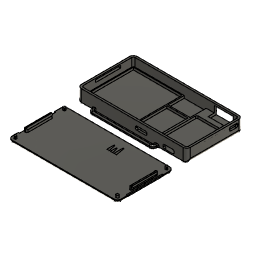
ArcturusV3 v8 (Autodesk Fusion 360 design; units mm, degrees)
Autodesk Fusion 360 part; units mm, degrees
(part 1 of 2)
sketch "Sketch8" plane through (0, 0, 0) normal (0, 0, 1) x (1, 0, 0)
  line L0 (45.1, 23.3) -> (-45.1, 23.3)
  line L1 (-45.1, -23.3) -> (45.1, -23.3)
  line L2 (45.1, -23.3) -> (45.1, 23.3)
  line L3 (45.1, 23.3) -> (-45.1, -23.3) construction
  line L4 (-45.1, 23.3) -> (45.1, -23.3) construction
  line L5 (-45.1, 23.3) -> (-46.1, 23.3)
  line L6 (-46.1, 23.3) -> (-46.1, -23.3)
  line L7 (-46.1, -23.3) -> (-45.1, -23.3)
  dimension "d32" = 90.2
  dimension "d33" = 46.6
  dimension "d223" = 1
  constraint horizontal L0
  constraint parallel L0 L1
  constraint coincident L3 origin
  constraint coincident L4 origin
  constraint horizontal L5
  constraint vertical L6
  constraint horizontal L7
  measures "d32" distance of L1.start L1.end
  measures "d33" distance of L0.end L1.start
  measures "d223" distance of L0.end L5.end
extrude "Extrude7" add sketch "Sketch8" along normal blind 10 makes body 1
fillet "Fillet4" radius 3 6 edges at (45.1, -23.3, 5) (45.1, 0, 0) (45.1, 23.3, 5) (-46.1, 23.3, 5) (-46.1, 0, 0) (-46.1, -23.3, 5) on bodies 1
sketch "Sketch13" plane through (0, 0, 10) normal (0, 0, 1) x (-1, 0, 0)
  line L0 (43.1, 23.3) -> (-42.1, 23.3)
  arc A0 (-42.1, 23.3) -> (-45.1, 20.3) centre (-42.1, 20.3) ccw
  line L1 (-45.1, 20.3) -> (-45.1, -20.3)
  arc A1 (-45.1, -20.3) -> (-42.1, -23.3) centre (-42.1, -20.3) ccw
  line L2 (-42.1, -23.3) -> (43.1, -23.3)
  line L3 (46.1, -20.3) -> (46.1, 20.3)
  arc A2 (46.1, 20.3) -> (43.1, 23.3) centre (43.1, 20.3) ccw
  arc A3 (43.1, -23.3) -> (46.1, -20.3) centre (43.1, -20.3) ccw
  line L4 (-43.5, 20.3) -> (-43.5, -20.3)
  arc A4 (-43.5, -20.3) -> (-42.1, -21.7) centre (-42.1, -20.3) ccw
  line L5 (-42.1, -21.7) -> (43.1, -21.7)
  arc A5 (43.1, -21.7) -> (44.5, -20.3) centre (43.1, -20.3) ccw
  line L6 (44.5, -20.3) -> (44.5, 20.3)
  arc A6 (44.5, 20.3) -> (43.1, 21.7) centre (43.1, 20.3) ccw
  line L7 (43.1, 21.7) -> (-42.1, 21.7)
  arc A7 (-42.1, 21.7) -> (-43.5, 20.3) centre (-42.1, 20.3) ccw
  dimension "d276" = -1.6
extrude "Extrude8" cut sketch "Sketch13" against normal blind 6 contours L4 A4 L5 A5 L6 A6 L7 A7 bodies 1
sketch "Sketch17" plane through (0, 0, 4) normal (0, 0, 1) x (-1, 0, 0)
  line L0 (1.989, 21.7) -> (-15.811, 21.7)
  line L1 (-15.811, 21.7) -> (-15.811, -6.1)
  line L2 (-14.811, -7.1) -> (0.989, -7.1)
  line L3 (1.989, -6.1) -> (1.989, 21.7)
  line L4 (1.989, -6.1) -> (1.989, -7.1)
  line L5 (1.989, -7.1) -> (0.989, -7.1)
  line L6 (-14.811, -7.1) -> (-15.811, -7.1)
  line L7 (-15.811, -6.1) -> (-15.811, -7.1)
  arc A0 (-42.1, 21.7) -> (-43.5, 20.3) centre (-42.1, 20.3) ccw
  line L8 (-43.5, 20.3) -> (-43.5, -20.3)
  arc A1 (-43.5, -20.3) -> (-42.1, -21.7) centre (-42.1, -20.3) ccw
  line L9 (-42.1, -21.7) -> (43.1, -21.7)
  arc A2 (43.1, -21.7) -> (44.5, -20.3) centre (43.1, -20.3) ccw
  line L10 (44.5, -20.3) -> (44.5, 20.3)
  arc A3 (44.5, 20.3) -> (43.1, 21.7) centre (43.1, 20.3) ccw
  line L11 (43.1, 21.7) -> (-42.1, 21.7)
  point P0 (1.989, -7.1)
  point P1 (43.1, -21.1)
  point P2 (43.1, -21.3)
  point P3 (43.1, -21.3)
  dimension "d53" = 17.8
  dimension "d54" = 28.8
  constraint horizontal L0
  constraint vertical L1
  constraint horizontal L2
  constraint vertical L3
  constraint coincident P0 L2
  constraint coincident P0 L3
  constraint coincident P0 L4.end
  constraint perpendicular L1 L6
  constraint perpendicular L6 L7
  measures "d53" distance of L0.start L0.end
  measures "d54" distance of L0.start P0
extrude "Extrude10" cut sketch "Sketch17" against normal blind 2 contours L0 L1 L2 L3 L4 L5 L6 L7 L11 bodies 1
sketch "Sketch20" plane through (0, 0, 4) normal (0, 0, 1) x (-1, 0, 0)
  line L0 (1.989, 21.7) -> (1.989, -7.1)
  line L1 (1.989, -7.1) -> (-15.811, -7.1)
  line L2 (-15.811, -7.1) -> (-15.811, 21.7)
  line L3 (-15.811, 21.7) -> (-42.1, 21.7)
  line L4 (43.1, 21.7) -> (1.989, 21.7)
  line L5 (1, -8) -> (-15.4, -8)
  line L6 (-16.4, -9) -> (-16.4, -21.4)
  line L7 (-16.4, -21.4) -> (2, -21.4)
  line L8 (2, -21.4) -> (2, -9)
  line L9 (-16.4, -9) -> (-16.4, -8)
  line L10 (-15.4, -8) -> (-16.4, -8)
  line L11 (1, -8) -> (2, -8)
  line L12 (2, -9) -> (2, -8)
  arc A0 (-42.1, 21.7) -> (-43.5, 20.3) centre (-42.1, 20.3) ccw
  line L13 (-43.5, 20.3) -> (-43.5, -20.3)
  arc A1 (-43.5, -20.3) -> (-42.1, -21.7) centre (-42.1, -20.3) ccw
  line L14 (-42.1, -21.7) -> (43.1, -21.7)
  arc A2 (43.1, -21.7) -> (44.5, -20.3) centre (43.1, -20.3) ccw
  line L15 (44.5, -20.3) -> (44.5, 20.3)
  arc A3 (44.5, 20.3) -> (43.1, 21.7) centre (43.1, 20.3) ccw
  point P0 (2, -8)
  point P1 (-16.4, -8)
  dimension "d61" = 18.4
  dimension "d62" = 13.4
  constraint horizontal L5
  constraint vertical L6
  constraint horizontal L7
  constraint vertical L8
  constraint coincident P1 L5
  constraint coincident P1 L6
  constraint coincident P0 L5
  constraint coincident P0 L8
  constraint coincident P1 L9.end
  constraint coincident P0 L11.end
  measures "d61" distance of P0 P1
  measures "d62" distance of P0 L7.end
extrude "Extrude11" cut sketch "Sketch20" against normal blind 2 contours L5 L6 L7 L8 L9 L10 L11 L12 bodies 1
sketch "Sketch24" plane through (0, 0, 4) normal (0, 0, 1) x (-1, 0, 0)
  line L0 (-16.4, -8) -> (2, -8)
  line L1 (2, -8) -> (2, -21.4)
  line L2 (2, -21.4) -> (-16.4, -21.4)
  line L3 (-16.4, -21.4) -> (-16.4, -8)
  line L4 (1.989, 21.7) -> (1.989, -7.1)
  line L5 (1.989, -7.1) -> (-15.811, -7.1)
  line L6 (-15.811, -7.1) -> (-15.811, 21.7)
  line L7 (-15.811, 21.7) -> (-42.1, 21.7)
  line L8 (43.1, 21.7) -> (1.989, 21.7)
  line L9 (4, 21) -> (43.5, 21)
  line L10 (43.5, 21) -> (43.5, -21)
  line L11 (43.5, -21) -> (4, -21)
  line L12 (3, -20) -> (3, 20)
  arc A0 (4, 21) -> (3, 20) centre (4, 20) ccw
  arc A1 (3, -20) -> (4, -21) centre (4, -20) ccw
  arc A2 (-42.1, 21.7) -> (-43.5, 20.3) centre (-42.1, 20.3) ccw
  line L13 (-43.5, 20.3) -> (-43.5, -20.3)
  arc A3 (-43.5, -20.3) -> (-42.1, -21.7) centre (-42.1, -20.3) ccw
  line L14 (-42.1, -21.7) -> (43.1, -21.7)
  arc A4 (43.1, -21.7) -> (44.5, -20.3) centre (43.1, -20.3) ccw
  line L15 (44.5, -20.3) -> (44.5, 20.3)
  arc A5 (44.5, 20.3) -> (43.1, 21.7) centre (43.1, 20.3) ccw
  point P0 (3, 21)
  point P1 (3, -21)
  dimension "d67" = 40.5
  dimension "d68" = 42
  dimension "d97" = 1
  constraint horizontal L9
  constraint vertical L10
  constraint horizontal L11
  constraint vertical L12
  constraint coincident P0 L9
  constraint coincident P0 L12
  constraint tangent L9 A0
  constraint tangent L12 A0
  constraint coincident P1 L11
  constraint coincident P1 L12
  constraint tangent L11 A1
  constraint tangent L12 A1
  constraint equal A0 A1
  measures "d67" distance of P0 L9.end
  measures "d68" distance of P0 P1
  measures "d97" radius of A0
extrude "Extrude12" cut sketch "Sketch24" against normal blind 2 contours L9 L10 L11 L12 A0 A1 bodies 1
sketch "Sketch26" plane through (0, 0, 4) normal (0, 0, 1) x (-1, 0, 0)
  line L0 (43.5, -21) -> (4, -21)
  line L1 (3, -20) -> (3, 20)
  line L2 (4, 21) -> (43.5, 21)
  line L3 (43.5, 21) -> (43.5, -21)
  line L4 (-15.811, 21.7) -> (-42.1, 21.7)
  line L5 (1.989, 21.7) -> (1.989, -7.1)
  line L6 (1.989, -7.1) -> (-15.811, -7.1)
  line L7 (-15.811, -7.1) -> (-15.811, 21.7)
  line L8 (-16.4, -8) -> (2, -8)
  line L9 (2, -8) -> (2, -21.4)
  line L10 (2, -21.4) -> (-16.4, -21.4)
  line L11 (-16.4, -21.4) -> (-16.4, -8)
  line L12 (-17.533, 21.7) -> (-42.933, 21.7)
  line L13 (-42.933, 21.7) -> (-42.933, -12.7)
  line L14 (-41.933, -13.7) -> (-18.533, -13.7)
  line L15 (-17.533, -12.7) -> (-17.533, 21.7)
  arc A0 (-18.533, -13.7) -> (-17.533, -12.7) centre (-18.533, -12.7) ccw
  arc A1 (-42.933, -12.7) -> (-41.933, -13.7) centre (-41.933, -12.7) ccw
  arc A2 (3, -20) -> (4, -21) centre (4, -20) ccw
  arc A3 (4, 21) -> (3, 20) centre (4, 20) ccw
  arc A4 (-42.1, 21.7) -> (-43.5, 20.3) centre (-42.1, 20.3) ccw
  line L16 (-43.5, 20.3) -> (-43.5, -20.3)
  arc A5 (-43.5, -20.3) -> (-42.1, -21.7) centre (-42.1, -20.3) ccw
  line L17 (-42.1, -21.7) -> (43.1, -21.7)
  arc A6 (43.1, -21.7) -> (44.5, -20.3) centre (43.1, -20.3) ccw
  line L18 (44.5, -20.3) -> (44.5, 20.3)
  arc A7 (44.5, 20.3) -> (43.1, 21.7) centre (43.1, 20.3) ccw
  line L19 (43.1, 21.7) -> (1.989, 21.7)
  point P0 (-17.533, -13.7)
  dimension "d73" = 25.4
  dimension "d74" = 35.4
  dimension "d94" = 1
  constraint horizontal L12
  constraint vertical L13
  constraint horizontal L14
  constraint vertical L15
  constraint coincident P0 L14
  constraint coincident P0 L15
  constraint tangent L14 A0
  constraint tangent L15 A0
  constraint tangent L13 A1
  constraint tangent L14 A1
  constraint equal A0 A1
  measures "d73" distance of L12.start L12.end
  measures "d74" distance of L12.start P0
  measures "d94" radius of A0
extrude "Extrude13" cut sketch "Sketch26" against normal blind 2 contours L4 L12 L13 L14 L15 A0 A1 A4 | L12 L13 A4 bodies 1
sketch "Sketch29" plane through (0, 0, 4) normal (0, 0, 1) x (-1, 0, 0)
  line L0 (-16.4, -8) -> (2, -8)
  line L1 (2, -8) -> (2, -21.4)
  line L2 (2, -21.4) -> (-16.4, -21.4)
  line L3 (-16.4, -21.4) -> (-16.4, -8)
  line L4 (-17.533, 21.7) -> (-17.533, -12.7)
  line L5 (-18.533, -13.7) -> (-41.933, -13.7)
  line L6 (-42.933, -12.7) -> (-42.933, 21.4252)
  line L7 (43.5, -21) -> (4, -21)
  line L8 (3, -20) -> (3, 20)
  line L9 (4, 21) -> (43.5, 21)
  line L10 (43.5, 21) -> (43.5, -21)
  line L11 (43.1, 21.7) -> (1.989, 21.7)
  line L12 (1.989, 21.7) -> (1.989, -7.1)
  line L13 (1.989, -7.1) -> (-15.811, -7.1)
  line L14 (-15.811, -7.1) -> (-15.811, 21.7)
  line L15 (-15.811, 21.7) -> (-17.533, 21.7)
  line L16 (-39.0432, -21.7) -> (-23.2432, -21.7)
  line L17 (-23.2432, -21.7) -> (-23.2432, -15.5)
  line L18 (-23.2432, -15.5) -> (-39.0432, -15.5)
  line L19 (-39.0432, -15.5) -> (-39.0432, -21.7)
  arc A0 (-18.533, -13.7) -> (-17.533, -12.7) centre (-18.533, -12.7) ccw
  arc A1 (-42.933, -12.7) -> (-41.933, -13.7) centre (-41.933, -12.7) ccw
  arc A2 (3, -20) -> (4, -21) centre (4, -20) ccw
  arc A3 (4, 21) -> (3, 20) centre (4, 20) ccw
  arc A4 (-42.933, 21.4252) -> (-43.5, 20.3) centre (-42.1, 20.3) ccw
  line L20 (-43.5, 20.3) -> (-43.5, -20.3)
  arc A5 (-43.5, -20.3) -> (-42.1, -21.7) centre (-42.1, -20.3) ccw
  line L21 (-42.1, -21.7) -> (43.1, -21.7)
  arc A6 (43.1, -21.7) -> (44.5, -20.3) centre (43.1, -20.3) ccw
  line L22 (44.5, -20.3) -> (44.5, 20.3)
  arc A7 (44.5, 20.3) -> (43.1, 21.7) centre (43.1, 20.3) ccw
  dimension "d81" = 15.8
  dimension "d82" = 6.2
  constraint horizontal L16
  constraint vertical L17
  constraint horizontal L18
  constraint vertical L19
  measures "d81" distance of L16.start L16.end
  measures "d82" distance of L16.start L18.end
extrude "Extrude14" cut sketch "Sketch29" against normal blind 2 contours L16 L17 L18 L19 L21 bodies 1
move_face "MoveFace1" by (0, -0.1, 0) 1 faces at (10.2667, 21.4, 3.3333) on bodies 1
move_face "MoveFace2" by (0, 0.3, 0) 1 faces at (10.2667, 21.3, 3.3333) on bodies 1
move_face "MoveFace3" by (0, 0.1, 0) 1 faces at (10.2667, 21.6, 3.3333) on bodies 1
sketch "Sketch31" plane through (0, 21.7, 0) normal (0, -1, 0) x (1, 0, 0)
  line L0 (-2, 4) -> (-2, 2)
  line L1 (-2, 2) -> (16.4, 2)
  line L2 (16.4, 2) -> (16.4, 4)
  line L3 (16.4, 4) -> (23.2432, 4)
  line L4 (23.2432, 4) -> (23.2432, 2)
  line L5 (23.2432, 2) -> (39.0432, 2)
  line L6 (39.0432, 2) -> (39.0432, 4)
  line L7 (39.0432, 4) -> (42.1, 4)
  line L8 (42.1, 10) -> (-43.1, 10)
  line L9 (23.2432, 2) -> (39.0432, 2)
  line L10 (39.0432, 2) -> (39.0432, 9.65)
  line L11 (39.0432, 9.65) -> (23.2432, 9.65)
  line L12 (23.2432, 9.65) -> (23.2432, 2)
  line L13 (42.1, 4) -> (42.1, 10)
  line L14 (-43.1, 10) -> (-43.1, 4)
  line L15 (-43.1, 4) -> (-2, 4)
  dimension "d85" = 15.8
  dimension "d86" = 7.65
  constraint horizontal L9
  constraint vertical L10
  constraint horizontal L11
  constraint vertical L12
  constraint coincident L4.end L5.start
  measures "d85" distance of L4.end L5.end
  measures "d86" distance of L4.end L11.end
extrude "Extrude15" cut sketch "Sketch31" against normal blind 2 contours L4 L5 L6 L9 L10 L11 L12 bodies 1
sketch "Sketch32" plane through (0, -21.7, 0) normal (0, 1, 0) x (-1, 0, 0)
  line L0 (43.1, 10) -> (-42.1, 10)
  line L1 (-42.933, 2) -> (-17.533, 2)
  line L2 (-17.533, 2) -> (-17.533, 4)
  line L3 (-17.533, 4) -> (-15.811, 4)
  line L4 (-15.811, 4) -> (-15.811, 2)
  line L5 (-15.811, 2) -> (1.989, 2)
  line L6 (1.989, 2) -> (1.989, 4)
  line L7 (1.989, 4) -> (43.1, 4)
  line L8 (-10.7121, 4.0287) -> (-3.2121, 4.0287)
  line L9 (-2.2121, 5.0287) -> (-2.2121, 6.0287)
  line L10 (-3.2121, 7.0287) -> (-10.7121, 7.0287)
  line L11 (-11.7121, 6.0287) -> (-11.7121, 5.0287)
  arc A0 (-10.7121, 7.0287) -> (-11.7121, 6.0287) centre (-10.7121, 6.0287) ccw
  arc A1 (-2.2121, 6.0287) -> (-3.2121, 7.0287) centre (-3.2121, 6.0287) ccw
  arc A2 (-3.2121, 4.0287) -> (-2.2121, 5.0287) centre (-3.2121, 5.0287) ccw
  arc A3 (-11.7121, 5.0287) -> (-10.7121, 4.0287) centre (-10.7121, 5.0287) ccw
  line L12 (-42.1, 10) -> (-42.1, 4)
  line L13 (-42.1, 4) -> (-42.933, 4)
  line L14 (-42.933, 4) -> (-42.933, 2)
  line L15 (43.1, 4) -> (43.1, 10)
  point P0 (-11.7121, 4.0287)
  point P1 (-2.2121, 4.0287)
  point P2 (-11.7121, 7.0287)
  dimension "d89" = 9.5
  dimension "d90" = 3
  dimension "d91" = 1
  constraint horizontal L8
  constraint vertical L9
  constraint horizontal L10
  constraint vertical L11
  constraint coincident P2 L10
  constraint coincident P2 L11
  constraint tangent L10 A0
  constraint tangent L11 A0
  constraint tangent L9 A1
  constraint tangent L10 A1
  constraint equal A0 A1
  constraint coincident P1 L8
  constraint coincident P1 L9
  constraint tangent L8 A2
  constraint tangent L9 A2
  constraint equal A0 A2
  constraint coincident P0 L8
  constraint coincident P0 L11
  constraint tangent L8 A3
  constraint tangent L11 A3
  constraint equal A0 A3
  measures "d89" distance of P0 P1
  measures "d90" distance of P0 P2
  measures "d91" radius of A0
extrude "Extrude16" cut sketch "Sketch32" against normal blind 2 contours L8 L9 L10 L11 A0 A1 A2 A3 bodies 1
sketch "Sketch33" plane through (0, -21.7, 0) normal (0, 1, 0) x (-1, 0, 0)
  line L0 (-3.2121, 4.0287) -> (-10.7121, 4.0287)
  arc A0 (-11.7121, 5.0287) -> (-10.7121, 4.0287) centre (-10.7121, 5.0287) ccw
  line L1 (-11.7121, 5.0287) -> (-11.7121, 6.0287)
  arc A1 (-10.7121, 7.0287) -> (-11.7121, 6.0287) centre (-10.7121, 6.0287) ccw
  line L2 (-10.7121, 7.0287) -> (-3.2121, 7.0287)
  arc A2 (-2.2121, 6.0287) -> (-3.2121, 7.0287) centre (-3.2121, 6.0287) ccw
  line L3 (-2.2121, 6.0287) -> (-2.2121, 5.0287)
  arc A3 (-3.2121, 4.0287) -> (-2.2121, 5.0287) centre (-3.2121, 5.0287) ccw
  line L4 (43.1, 10) -> (-42.1, 10)
  line L5 (-42.933, 2) -> (-17.533, 2)
  line L6 (-17.533, 2) -> (-17.533, 4)
  line L7 (-17.533, 4) -> (-15.811, 4)
  line L8 (-15.811, 4) -> (-15.811, 2)
  line L9 (-15.811, 2) -> (1.989, 2)
  line L10 (1.989, 2) -> (1.989, 4)
  line L11 (1.989, 4) -> (43.1, 4)
  line L12 (-33.5451, 2) -> (-26.3451, 2)
  line L13 (-25.3451, 3) -> (-25.3451, 4.2)
  line L14 (-26.3451, 5.2) -> (-33.5451, 5.2)
  line L15 (-34.5451, 4.2) -> (-34.5451, 3)
  arc A4 (-33.5451, 5.2) -> (-34.5451, 4.2) centre (-33.5451, 4.2) ccw
  arc A5 (-25.3451, 4.2) -> (-26.3451, 5.2) centre (-26.3451, 4.2) ccw
  arc A6 (-26.3451, 2) -> (-25.3451, 3) centre (-26.3451, 3) ccw
  arc A7 (-34.5451, 3) -> (-33.5451, 2) centre (-33.5451, 3) ccw
  line L16 (-42.1, 10) -> (-42.1, 4)
  line L17 (-42.1, 4) -> (-42.933, 4)
  line L18 (-42.933, 4) -> (-42.933, 2)
  line L19 (43.1, 4) -> (43.1, 10)
  point P0 (-34.5451, 2)
  point P1 (-25.3451, 2)
  point P2 (-34.5451, 5.2)
  dimension "d98" = 9.2
  dimension "d99" = 3.2
  dimension "d100" = 1
  dimension "d101" = 1
  constraint horizontal L12
  constraint vertical L13
  constraint horizontal L14
  constraint vertical L15
  constraint coincident L5 P0
  constraint coincident P2 L14
  constraint coincident P2 L15
  constraint tangent L14 A4
  constraint tangent L15 A4
  constraint tangent L13 A5
  constraint tangent L14 A5
  constraint coincident P1 L12
  constraint coincident P1 L13
  constraint tangent L12 A6
  constraint tangent L13 A6
  constraint equal A5 A6
  constraint coincident P0 L12
  constraint coincident P0 L15
  constraint tangent L12 A7
  constraint tangent L15 A7
  constraint equal A5 A7
  measures "d98" distance of P0 P1
  measures "d99" distance of P0 P2
  measures "d100" radius of A4
  measures "d101" radius of A5
extrude "Extrude17" cut sketch "Sketch33" against normal blind 2 contours L5 L12 L13 L14 L15 A4 A5 A6 A7 bodies 1
sketch "Sketch36" plane through (0, 0, 0) normal (0, 0, 1) x (1, 0, 0)
  line L0 (-33, -23) -> (-33, -24.5)
  line L1 (-30, -27.5) -> (18, -27.5)
  line L2 (21, -24.5) -> (21, -23)
  line L3 (-33, -23) -> (21, -23)
  arc A0 (18, -27.5) -> (21, -24.5) centre (18, -24.5) ccw
  arc A1 (-33, -24.5) -> (-30, -27.5) centre (-30, -24.5) ccw
  line L4 (21, -24.5) -> (21, -23)
  line L5 (21, -23) -> (18, -23)
  point P0 (21, -27.5)
  dimension "d111" = 3
  constraint vertical L0
  constraint horizontal L1
  constraint vertical L2
  constraint coincident P0 L1
  constraint coincident P0 L2
  constraint tangent L1 A0
  constraint tangent L2 A0
  constraint tangent L0 A1
  constraint tangent L1 A1
  constraint equal A0 A1
  constraint vertical L4
  constraint horizontal L5
  measures "d111" radius of A0
extrude "Extrude1" add sketch "Sketch36" along normal blind 3 separate body makes body 2 in component "Component"
sketch "Sketch38" plane through (0, 0, 3) normal (0, 0, 1) x (-1, 0, 0)
  line L0 (33, 23) -> (33, 24.5)
  arc A0 (33, 24.5) -> (30, 27.5) centre (30, 24.5) ccw
  line L1 (30, 27.5) -> (-18, 27.5)
  arc A1 (-18, 27.5) -> (-21, 24.5) centre (-18, 24.5) ccw
  line L2 (-21, 24.5) -> (-21, 23)
  line L3 (-21, 23) -> (33, 23)
  line L4 (30, 25.5) -> (-17.866, 25.5)
  line L5 (30.866, 24.5) -> (30.866, 23)
  line L6 (30.866, 23) -> (-18.866, 23)
  line L7 (-18.866, 23) -> (-18.866, 24.5)
  line L8 (-17.866, 25.5) -> (29.866, 25.5)
  line L9 (-18.866, 24.5) -> (-18.866, 23)
  arc A2 (-17.866, 25.5) -> (-18.866, 24.5) centre (-17.866, 24.5) ccw
  line L10 (30.866, 24.5) -> (30.866, 23)
  arc A3 (30.866, 24.5) -> (29.866, 25.5) centre (29.866, 24.5) ccw
  dimension "d273" = 1
  dimension "d274" = 1
  constraint vertical L5
  constraint horizontal L6
  constraint vertical L7
  constraint coincident L3 L5.end
  constraint tangent L9 A2
  constraint tangent L8 A2
  constraint perpendicular L6 L10
  constraint tangent L8 A3
  constraint tangent L5 A3
  measures "d273" radius of A2
  measures "d274" radius of A3
extrude "Extrude3" cut sketch "Sketch38" against normal blind 3 contours L3 L4 L5 L6 L7 L8 L9 A2 L10 A3 bodies 2 in component "Component"
combine "Combine2" operation add target body 1 tool bodies 2 2 body 2 seen with x (1, 0, 0) y (0, 1, 0) z (0, 0, 1) at (0, 0, 0) body 2 seen with x (-1, 0, 0) y (0, -1, 0) z (0, 0, 1) at (-12, 0, 0)
move_face "MoveFace4" by (0, 0, 1) 1 faces at (-14.7, 22.7667, 10) on bodies 1
sketch "Sketch40" plane through (43.5, 0, 0) normal (-1, 0, 0) x (0, -1, 0)
  line L0 (-18.5, 9) -> (-13.5, 9)
  line L1 (-12.5, 8) -> (-12.5, 7)
  line L2 (-13.5, 6) -> (-18.5, 6)
  line L3 (-19.5, 7) -> (-19.5, 8)
  arc A0 (-18.5, 9) -> (-19.5, 8) centre (-18.5, 8) ccw
  arc A1 (-13.5, 6) -> (-12.5, 7) centre (-13.5, 7) ccw
  arc A2 (-12.5, 8) -> (-13.5, 9) centre (-13.5, 8) ccw
  arc A3 (-19.5, 7) -> (-18.5, 6) centre (-18.5, 7) ccw
  line L4 (20.3, 11) -> (-20.3, 11)
  line L5 (-20.3, 11) -> (-20.3, 4)
  line L6 (-20.3, 4) -> (20.3, 4)
  line L7 (20.3, 4) -> (20.3, 11)
  dimension "d121" = 1
  constraint horizontal L0
  constraint vertical L1
  constraint horizontal L2
  constraint vertical L3
  constraint tangent L0 A0
  constraint tangent L3 A0
  constraint tangent L1 A1
  constraint tangent L2 A1
  constraint equal A0 A1
  constraint tangent L0 A2
  constraint tangent L1 A2
  constraint equal A0 A2
  constraint tangent L2 A3
  constraint tangent L3 A3
  constraint equal A0 A3
  measures "d121" radius of A0
extrude "Extrude18" cut sketch "Sketch40" against normal blind 2 contours L0 L1 L2 L3 A0 A1 A2 A3 bodies 1
fillet "Fillet6" radius 1 32 edges at (44.2213, 22.4213, 0.8787) (31.55, 23.3, 0) (21, 23.9, 0) (20.1213, 26.6213, 0) (-6, 27.5, 0) (-32.1213, 26.6213, 0) (-33, 23.9, 0) (21, 23.9, 3) (20.1213, 26.6213, 3) (-6, 27.5, 3) (-32.1213, 26.6213, 3) (-33, 23.9, 3) (-33, 23.3, 1.5) (21, 23.3, 1.5) (-38.05, 23.3, 0) (-45.2213, 22.4213, 0.8787) (-45.2213, -22.4213, 0.8787) (-38.05, -23.3, 0) (-33, -23.3, 1.5) (-33, -23.9, 0) (-32.1213, -26.6213, 0) (-6, -27.5, 0) (20.1213, -26.6213, 0) (21, -23.9, 0) (-33, -23.9, 3) (-32.1213, -26.6213, 3) (-6, -27.5, 3) (20.1213, -26.6213, 3) (21, -23.9, 3) (31.55, -23.3, 0) (44.2213, -22.4213, 0.8787) (21, -23.3, 1.5) on bodies 1
sketch "Sketch41" plane through (0, 0, 0) normal (0, 0, 1) x (1, 0, 0)
  line L0 (-43.1, 38.7) -> (42.1, 38.7)
  line L1 (45.1, 41.7) -> (45.1, 82.3)
  line L2 (42.1, 85.3) -> (-43.1, 85.3)
  line L3 (-46.1, 82.3) -> (-46.1, 41.7)
  line L4 (-46.1, 38.7) -> (45.1, 85.3) construction
  line L5 (45.1, 38.7) -> (-46.1, 85.3) construction
  arc A0 (42.1, 38.7) -> (45.1, 41.7) centre (42.1, 41.7) ccw
  arc A1 (-46.1, 41.7) -> (-43.1, 38.7) centre (-43.1, 41.7) ccw
  arc A2 (-43.1, 85.3) -> (-46.1, 82.3) centre (-43.1, 82.3) ccw
  arc A3 (45.1, 82.3) -> (42.1, 85.3) centre (42.1, 82.3) ccw
  point P0 (-0.5, 62)
  dimension "d126" = 91.2
  dimension "d127" = 46.6
  dimension "d128" = 3
  constraint horizontal L0
  constraint perpendicular L0 L1
  constraint parallel L0 L2
  constraint parallel L1 L3
  constraint coincident L4 P0
  constraint coincident L5 P0
  constraint coincident L5.start L1
  constraint coincident L5.start L0
  constraint tangent L1 A0
  constraint tangent L0 A0
  constraint coincident L4.start L3
  constraint coincident L4.start L0
  constraint tangent L3 A1
  constraint tangent L0 A1
  constraint equal A0 A1
  constraint coincident L5.end L2
  constraint coincident L5.end L3
  constraint tangent L2 A2
  constraint tangent L3 A2
  constraint equal A0 A2
  constraint coincident L4.end L2
  constraint coincident L4.end L1
  constraint tangent L2 A3
  constraint tangent L1 A3
  constraint equal A0 A3
  measures "d126" distance of L4.end L5.end
  measures "d127" distance of L5.start L4.end
  measures "d128" radius of A0
extrude "Extrude19" add sketch "Sketch41" along normal blind 2.5 separate body makes body 3
move_body "Move4" bodies 3 to x (1, 0, 0) y (0, 1, 0) z (0, 0, 1) at (0, -63, 11)
move_body "Move5" bodies 3 to x (1, 0, 0) y (0, 1, 0) z (0, 0, 1) at (0, 0, 10)
sketch "Sketch48" plane through (43.5, 0, 0) normal (-1, 0, 0) x (0, -1, 0)
  line L0 (-19.5, 7) -> (-19.5, 8)
  arc A0 (-18.5, 9) -> (-19.5, 8) centre (-18.5, 8) ccw
  line L1 (-18.5, 9) -> (-13.5, 9)
  arc A1 (-12.5, 8) -> (-13.5, 9) centre (-13.5, 8) ccw
  line L2 (-12.5, 8) -> (-12.5, 7)
  arc A2 (-13.5, 6) -> (-12.5, 7) centre (-13.5, 7) ccw
  line L3 (-13.5, 6) -> (-18.5, 6)
  arc A3 (-19.5, 7) -> (-18.5, 6) centre (-18.5, 7) ccw
  line L4 (20.3, 11) -> (-20.3, 11)
  line L5 (-20.3, 11) -> (-20.3, 4)
  line L6 (-20.3, 4) -> (20.3, 4)
  line L7 (20.3, 4) -> (20.3, 11)
  line L8 (-20.3, 11) -> (-11, 11)
  line L9 (-11, 11) -> (-11, 10)
  line L10 (-11, 10) -> (-20.3, 10)
  line L11 (-20.3, 10) -> (-20.3, 11)
  line L12 (20.3, 11) -> (11, 11)
  line L13 (11, 11) -> (11, 10)
  line L14 (11, 10) -> (20.3, 10)
  line L15 (20.3, 10) -> (20.3, 11)
  line L16 (-11, 10) -> (11, 10)
  line L17 (11, 10) -> (11, 8)
  line L18 (11, 8) -> (-11, 8)
  line L19 (-11, 8) -> (-11, 10)
  line L20 (-19.5, 7) -> (-19.5, 8)
  arc A4 (-18.5, 9) -> (-19.5, 8) centre (-18.5, 8) ccw
  line L21 (-18.5, 9) -> (-13.5, 9)
  arc A5 (-12.5, 8) -> (-13.5, 9) centre (-13.5, 8) ccw
  line L22 (-12.5, 8) -> (-12.5, 7)
  arc A6 (-13.5, 6) -> (-12.5, 7) centre (-13.5, 7) ccw
  line L23 (-13.5, 6) -> (-18.5, 6)
  arc A7 (-19.5, 7) -> (-18.5, 6) centre (-18.5, 7) ccw
  line L24 (20.3, 11) -> (-20.3, 11)
  line L25 (-20.3, 11) -> (-20.3, 4)
  line L26 (-20.3, 4) -> (20.3, 4)
  line L27 (20.3, 4) -> (20.3, 11)
  constraint horizontal L8
  constraint vertical L9
  constraint horizontal L10
  constraint vertical L11
  constraint coincident L4.end L5.start
  constraint horizontal L12
  constraint vertical L13
  constraint horizontal L14
  constraint vertical L15
  constraint coincident L4.start L7.end
  constraint horizontal L16
  constraint vertical L17
  constraint horizontal L18
  constraint vertical L19
extrude "Extrude22" cut sketch "Sketch48" against normal blind 1 draft -45 contours L16 L17 L18 L19 bodies 1
sketch "Sketch49" plane through (-43.5, 0, 0) normal (1, 0, 0) x (0, 1, 0)
  line L0 (21, 4) -> (-21, 4)
  line L1 (-21, 4) -> (-21, 2)
  line L2 (-21, 2) -> (21, 2)
  line L3 (21, 2) -> (21, 4)
  line L4 (-21.3, 11) -> (-11, 11)
  line L5 (-11, 11) -> (-11, 10)
  line L6 (-11, 10) -> (-21.3, 10)
  line L7 (-21.3, 10) -> (-21.3, 11)
  line L8 (21.3, 11) -> (11, 11)
  line L9 (11, 11) -> (11, 10)
  line L10 (11, 10) -> (21.3, 10)
  line L11 (21.3, 10) -> (21.3, 11)
  line L12 (-11, 10) -> (11, 10)
  line L13 (11, 10) -> (11, 8)
  line L14 (11, 8) -> (-11, 8)
  line L15 (-11, 8) -> (-11, 10)
  constraint horizontal L4
  constraint vertical L5
  constraint horizontal L6
  constraint vertical L7
  constraint horizontal L8
  constraint vertical L9
  constraint horizontal L10
  constraint vertical L11
  constraint horizontal L12
  constraint vertical L13
  constraint horizontal L14
  constraint vertical L15
sketch "Sketch50" plane through (0, 0, 23.5) normal (0, 0, 1) x (-1, 0, 0)
  arc A0 (-45.1, -19.3) -> (-42.1, -22.3) centre (-42.1, -19.3) ccw
  line L0 (-42.1, -22.3) -> (43.1, -22.3)
  arc A1 (43.1, -22.3) -> (46.1, -19.3) centre (43.1, -19.3) ccw
  line L1 (46.1, -19.3) -> (46.1, 21.3)
  arc A2 (46.1, 21.3) -> (43.1, 24.3) centre (43.1, 21.3) ccw
  line L2 (43.1, 24.3) -> (-42.1, 24.3)
  arc A3 (-42.1, 24.3) -> (-45.1, 21.3) centre (-42.1, 21.3) ccw
  line L3 (-45.1, 21.3) -> (-45.1, -19.3)
  line L4 (46.1, -19.3) -> (44.1, -19.3)
  line L5 (44.1, -19.3) -> (44.1, -9)
  line L6 (44.1, -9) -> (46.1, -9)
  line L7 (46.1, -9) -> (46.1, -19.3)
  line L8 (46.1, 21.3) -> (44.1, 21.3)
  line L9 (44.1, 21.3) -> (44.1, 11)
  line L10 (44.1, 11) -> (46.1, 11)
  line L11 (46.1, 11) -> (46.1, 21.3)
  line L12 (44.1, -9) -> (46.1, -9)
  line L13 (46.1, -9) -> (46.1, 11)
  line L14 (46.1, 11) -> (44.1, 11)
  line L15 (44.1, 11) -> (44.1, -9)
  dimension "d143" = 2
  dimension "d144" = 10.3
  dimension "d145" = 2
  dimension "d146" = 10.3
  constraint horizontal L4
  constraint vertical L5
  constraint horizontal L6
  constraint vertical L7
  constraint coincident A1.end L1.start
  constraint horizontal L8
  constraint vertical L9
  constraint horizontal L10
  constraint vertical L11
  constraint coincident L1.end A2.start
  constraint horizontal L12
  constraint vertical L13
  constraint horizontal L14
  constraint vertical L15
  measures "d143" distance of A1.end L4.end
  measures "d144" distance of A1.end L6.end
  measures "d145" distance of L1.end L8.end
  measures "d146" distance of L1.end L10.end
sketch "Sketch53" plane through (0, 0, 23.5) normal (0, 0, 1) x (-1, 0, 0)
  arc A0 (46.1, 21.3) -> (43.1, 24.3) centre (43.1, 21.3) ccw
  line L0 (43.1, 24.3) -> (-42.1, 24.3)
  arc A1 (-42.1, 24.3) -> (-45.1, 21.3) centre (-42.1, 21.3) ccw
  line L1 (-45.1, 21.3) -> (-45.1, -19.3)
  arc A2 (-45.1, -19.3) -> (-42.1, -22.3) centre (-42.1, -19.3) ccw
  line L2 (-42.1, -22.3) -> (43.1, -22.3)
  arc A3 (43.1, -22.3) -> (46.1, -19.3) centre (43.1, -19.3) ccw
  line L3 (46.1, -19.3) -> (46.1, 21.3)
  line L4 (-45.1, -19.3) -> (-43.1, -19.3)
  line L5 (-43.1, -19.3) -> (-43.1, -9)
  line L6 (-43.1, -9) -> (-45.1, -9)
  line L7 (-45.1, -9) -> (-45.1, -19.3)
  line L8 (-45.1, 21.3) -> (-43.1, 21.3)
  line L9 (-43.1, 21.3) -> (-43.1, 11)
  line L10 (-43.1, 11) -> (-45.1, 11)
  line L11 (-45.1, 11) -> (-45.1, 21.3)
  line L12 (-43.1, -9) -> (-45.1, -9)
  line L13 (-45.1, -9) -> (-45.1, 11)
  line L14 (-45.1, 11) -> (-43.1, 11)
  line L15 (-43.1, 11) -> (-43.1, -9)
  line L16 (-43.1, 11) -> (-41.1, 11)
  line L17 (-41.1, 11) -> (-41.1, -11)
  line L18 (-41.1, -11) -> (-43.1, -11)
  line L19 (-43.1, -11) -> (-43.1, 11)
  dimension "d155" = 2
  dimension "d156" = 10.3
  dimension "d157" = 2
  dimension "d158" = 10.3
  dimension "d163" = 2
  dimension "d164" = 22
  constraint horizontal L4
  constraint vertical L5
  constraint horizontal L6
  constraint vertical L7
  constraint coincident L1.end A2.start
  constraint horizontal L8
  constraint vertical L9
  constraint horizontal L10
  constraint vertical L11
  constraint coincident A1.end L1.start
  constraint horizontal L12
  constraint vertical L13
  constraint horizontal L14
  constraint vertical L15
  constraint horizontal L16
  constraint vertical L17
  constraint horizontal L18
  constraint vertical L19
  measures "d155" distance of L1.end L4.end
  measures "d156" distance of L1.end L6.end
  measures "d157" distance of A1.end L8.end
  measures "d158" distance of A1.end L10.end
  measures "d163" distance of L9.end L16.end
  measures "d164" distance of L9.end L18.end
extrude "Extrude28" add sketch "Sketch53" along normal blind 3 contours L5 L15 L16 L17 L18 L19 bodies 3
sketch "Sketch56" plane through (0, 0, 23.5) normal (0, 0, 1) x (-1, 0, 0)
  line L0 (-43.1, 11) -> (-41.1, 11)
  line L1 (-41.1, 11) -> (-41.1, -11)
  line L2 (-41.1, -11) -> (-43.1, -11)
  arc A0 (-45.1, -19.3) -> (-42.1, -22.3) centre (-42.1, -19.3) ccw
  line L3 (-42.1, -22.3) -> (43.1, -22.3)
  arc A1 (43.1, -22.3) -> (46.1, -19.3) centre (43.1, -19.3) ccw
  line L4 (46.1, -19.3) -> (46.1, 21.3)
  arc A2 (46.1, 21.3) -> (43.1, 24.3) centre (43.1, 21.3) ccw
  line L5 (43.1, 24.3) -> (-42.1, 24.3)
  arc A3 (-42.1, 24.3) -> (-45.1, 21.3) centre (-42.1, 21.3) ccw
  line L6 (-45.1, 21.3) -> (-45.1, -19.3)
  line L7 (46.1, 21.3) -> (44.1, 21.3)
  line L8 (44.1, 21.3) -> (44.1, 11)
  line L9 (44.1, 11) -> (46.1, 11)
  line L10 (46.1, 11) -> (46.1, 21.3)
  line L11 (46.1, -19.3) -> (44.1, -19.3)
  line L12 (44.1, -19.3) -> (44.1, -9)
  line L13 (44.1, -9) -> (46.1, -9)
  line L14 (46.1, -9) -> (46.1, -19.3)
  line L15 (44.1, 13) -> (44.1, -9)
  line L16 (44.1, -9) -> (42.1, -9)
  line L17 (42.1, -9) -> (42.1, 13)
  line L18 (42.1, 13) -> (44.1, 13)
  line L19 (44.1, 13) -> (44.1, -9)
  line L20 (-43.1, -11) -> (-43.1, 11)
  dimension "d169" = 2
  dimension "d170" = 10.3
  dimension "d171" = 2
  dimension "d172" = 10.3
  dimension "d174" = 2
  dimension "d175" = 22
  constraint horizontal L7
  constraint vertical L8
  constraint horizontal L9
  constraint vertical L10
  constraint coincident L4.end A2.start
  constraint horizontal L11
  constraint vertical L12
  constraint horizontal L13
  constraint vertical L14
  constraint coincident A1.end L4.start
  constraint vertical L15
  constraint horizontal L16
  constraint vertical L17
  constraint horizontal L18
  constraint vertical L19
  measures "d169" distance of L4.end L7.end
  measures "d170" distance of L4.end L9.end
  measures "d171" distance of A1.end L11.end
  measures "d172" distance of A1.end L13.end
  measures "d174" distance of L12.end L16.end
  measures "d175" distance of L12.end L15.start
extrude "Extrude30" add sketch "Sketch56" along normal blind 3 contours L8 L15 L16 L17 L18 L19 bodies 3
move_body "Move6" bodies 3 to x (1, 0, 0) y (0, 1, 0) z (0, 0, 1) at (0, -55, -21)
sketch "Sketch58" plane through (0, 0, 2.5) normal (0, 0, 1) x (-1, 0, 0)
  line L0 (44.1, 46) -> (42.1, 46)
  line L1 (42.1, 46) -> (42.1, 68)
  line L2 (42.1, 68) -> (44.1, 68)
  line L3 (-43.1, 66) -> (-41.1, 66)
  line L4 (-41.1, 66) -> (-41.1, 44)
  line L5 (-41.1, 44) -> (-43.1, 44)
  arc A0 (-45.1, 35.7) -> (-42.1, 32.7) centre (-42.1, 35.7) ccw
  line L6 (-42.1, 32.7) -> (43.1, 32.7)
  arc A1 (43.1, 32.7) -> (46.1, 35.7) centre (43.1, 35.7) ccw
  line L7 (46.1, 35.7) -> (46.1, 76.3)
  arc A2 (46.1, 76.3) -> (43.1, 79.3) centre (43.1, 76.3) ccw
  line L8 (43.1, 79.3) -> (-42.1, 79.3)
  arc A3 (-42.1, 79.3) -> (-45.1, 76.3) centre (-42.1, 76.3) ccw
  line L9 (-45.1, 76.3) -> (-45.1, 35.7)
  line L10 (-45.1, 35.7) -> (-43.1, 35.7)
  line L11 (-43.1, 35.7) -> (-43.1, 41)
  line L12 (-43.1, 41) -> (-45.1, 41)
  line L13 (-45.1, 41) -> (-45.1, 35.7)
  line L14 (-45.1, 76.3) -> (-43.1, 76.3)
  line L15 (-43.1, 76.3) -> (-43.1, 71)
  line L16 (-43.1, 71) -> (-45.1, 71)
  line L17 (-45.1, 71) -> (-45.1, 76.3)
  line L18 (-45.1, 41) -> (-44.1, 41)
  line L19 (-44.1, 41) -> (-44.1, 71)
  line L20 (-44.1, 71) -> (-45.1, 71)
  line L21 (-45.1, 71) -> (-45.1, 41)
  line L22 (-43.1, 44) -> (-43.1, 66)
  line L23 (44.1, 68) -> (44.1, 46)
  dimension "d184" = 5.3
  dimension "d185" = 5.3
  constraint horizontal L10
  constraint vertical L11
  constraint horizontal L12
  constraint vertical L13
  constraint coincident A0.start L9.end
  constraint horizontal L14
  constraint vertical L15
  constraint horizontal L16
  constraint vertical L17
  constraint coincident A3.end L9.start
  constraint horizontal L18
  constraint vertical L19
  constraint horizontal L20
  constraint vertical L21
  constraint midpoint L16 L19.end
  measures "d184" distance of A0.start L12.end
  measures "d185" distance of A3.end L16.end
extrude "Extrude32" cut sketch "Sketch58" against normal blind 1 contours L9 L12 L16 L18 L19 L20 L21 bodies 3
sketch "Sketch59" plane through (0, 0, 2.5) normal (0, 0, 1) x (-1, 0, 0)
  line L0 (-44.1, 41) -> (-45.1, 41)
  line L1 (-45.1, 41) -> (-45.1, 35.7)
  arc A0 (-45.1, 35.7) -> (-42.1, 32.7) centre (-42.1, 35.7) ccw
  line L2 (-42.1, 32.7) -> (43.1, 32.7)
  arc A1 (43.1, 32.7) -> (46.1, 35.7) centre (43.1, 35.7) ccw
  line L3 (46.1, 35.7) -> (46.1, 76.3)
  arc A2 (46.1, 76.3) -> (43.1, 79.3) centre (43.1, 76.3) ccw
  line L4 (43.1, 79.3) -> (-42.1, 79.3)
  arc A3 (-42.1, 79.3) -> (-45.1, 76.3) centre (-42.1, 76.3) ccw
  line L5 (-45.1, 76.3) -> (-45.1, 71)
  line L6 (-45.1, 71) -> (-44.1, 71)
  line L7 (-44.1, 71) -> (-44.1, 41)
  line L8 (44.1, 46) -> (42.1, 46)
  line L9 (42.1, 46) -> (42.1, 68)
  line L10 (42.1, 68) -> (44.1, 68)
  line L11 (-43.1, 66) -> (-41.1, 66)
  line L12 (-41.1, 66) -> (-41.1, 44)
  line L13 (-41.1, 44) -> (-43.1, 44)
  line L14 (46.1, 76.3) -> (44.1, 76.3)
  line L15 (44.1, 76.3) -> (44.1, 71)
  line L16 (44.1, 71) -> (46.1, 71)
  line L17 (46.1, 71) -> (46.1, 76.3)
  line L18 (46.1, 35.7) -> (44.1, 35.7)
  line L19 (44.1, 35.7) -> (44.1, 41)
  line L20 (44.1, 41) -> (46.1, 41)
  line L21 (46.1, 41) -> (46.1, 35.7)
  line L22 (46.1, 71) -> (45.1, 71)
  line L23 (45.1, 71) -> (45.1, 41)
  line L24 (45.1, 41) -> (46.1, 41)
  line L25 (46.1, 41) -> (46.1, 71)
  line L26 (-43.1, 44) -> (-43.1, 66)
  line L27 (44.1, 68) -> (44.1, 46)
  dimension "d188" = 2
  dimension "d189" = 5.3
  dimension "d190" = 2
  dimension "d191" = 5.3
  constraint horizontal L14
  constraint vertical L15
  constraint horizontal L16
  constraint vertical L17
  constraint coincident L3.end A2.start
  constraint horizontal L18
  constraint vertical L19
  constraint horizontal L20
  constraint vertical L21
  constraint coincident A1.end L3.start
  constraint horizontal L22
  constraint vertical L23
  constraint horizontal L24
  constraint vertical L25
  constraint midpoint L20 L23.end
  measures "d188" distance of L3.end L14.end
  measures "d189" distance of L3.end L16.end
  measures "d190" distance of A1.end L18.end
  measures "d191" distance of A1.end L20.end
extrude "Extrude33" cut sketch "Sketch59" against normal blind 1 contours L3 L16 L20 L22 L23 L24 L25 bodies 3
fillet "Fillet7" radius 2 8 edges at (-0.5, -79.3, 0) (44.2213, -78.4213, 0) (45.1, -56, 0) (44.2213, -33.5787, 0) (-0.5, -32.7, 0) (-45.2213, -33.5787, 0) (-46.1, -56, 0) (-45.2213, -78.4213, 0) on bodies 3
fillet "Fillet8" radius 1 6 edges at (-42.1, -68, 4) (-42.1, -46, 4) (-42.1, -57, 5.5) (41.1, -55, 5.5) (41.1, -66, 4) (41.1, -44, 4) on bodies 3
sketch "Sketch61" plane through (43.1, 0, 0) normal (1, 0, 0) x (0, 1, 0)
  line L0 (-66, 2.5) -> (-44, 2.5)
  line L1 (-44, 2.5) -> (-44, 5.5)
  line L2 (-44, 5.5) -> (-66, 5.5)
  line L3 (-66, 5.5) -> (-66, 2.5)
  line L4 (-65.8, 2.7) -> (-44.2, 2.7)
  line L5 (-44.2, 2.7) -> (-44.2, 5.3)
  line L6 (-44.2, 5.3) -> (-65.8, 5.3)
  line L7 (-65.8, 5.3) -> (-65.8, 2.7)
  dimension "d204" = -0.2
extrude "Extrude34" add sketch "Sketch61" along normal blind 0.8 draft -45 contours L4 L5 L6 L7 bodies 3
sketch "Sketch62" plane through (-44.1, 0, 0) normal (-1, 0, 0) x (0, -1, 0)
  line L0 (46, 2.5) -> (68, 2.5)
  line L1 (68, 2.5) -> (68, 5.5)
  line L2 (68, 5.5) -> (46, 5.5)
  line L3 (46, 5.5) -> (46, 2.5)
  line L4 (46.2, 2.7) -> (67.8, 2.7)
  line L5 (67.8, 2.7) -> (67.8, 5.3)
  line L6 (67.8, 5.3) -> (46.2, 5.3)
  line L7 (46.2, 5.3) -> (46.2, 2.7)
  dimension "d207" = -0.2
extrude "Extrude35" add sketch "Sketch62" along normal blind 0.8 draft -45 contours L4 L5 L6 L7 bodies 3
sketch "Sketch65" plane through (0, 0, 0) normal (0, 0, 1) x (1, 0, 0)
  line L0 (-31.5, -75.5) -> (-36.102, -62.8561)
  line L1 (-33.75, -75.5) -> (-31.5, -75.5)
  line L2 (-42.75, -75.5) -> (-40.95, -75.5)
  line L3 (-37.4232, -69.8585) -> (-35.6232, -69.8585)
  line L4 (-37.8902, -68.4523) -> (-36.0902, -68.4523)
  line L5 (-37.9483, -62.8561) -> (-36.0902, -68.4523)
  line L6 (-35.6232, -69.8585) -> (-33.75, -75.5)
  line L7 (-39.6549, -71.2689) -> (-42.1421, -73.5164)
  line L8 (-39.6549, -71.2689) -> (-40.4312, -67.9335)
  line L9 (-39.6549, -71.2689) -> (-40.4312, -67.9335)
  line L10 (-40.189, -67.6451) -> (-39.4793, -70.6952)
  line L11 (-42.3179, -74.0901) -> (-39.8305, -71.8426)
  line L12 (-40.95, -75.5) -> (-39.8305, -71.8426)
  line L13 (-40.4312, -67.9335) -> (-42.1421, -73.5164)
  line L14 (-42.3179, -74.0901) -> (-42.75, -75.5)
  line L15 (-38.3598, -67.0378) -> (-40.189, -67.6451)
  line L16 (-40.2554, -67.3599) -> (-38.4517, -66.761)
  line L17 (-39.2942, -64.2237) -> (-40.35, -67.1)
  line L18 (-40.35, -67.1) -> (-40.2554, -67.3599)
  line L19 (-38.3598, -67.0378) -> (-39.15, -70.4)
  line L20 (-39.15, -70.4) -> (-39.4793, -70.6952)
  line L21 (-39.2942, -64.2237) -> (-39.1328, -63.7838)
  line L22 (-39.1328, -63.7838) -> (-38.7923, -62.8561)
  line L23 (-38.7923, -62.8561) -> (-38.4517, -66.761)
  line L24 (-37.1611, -69.8585) -> (-38.1351, -69.8585)
  line L25 (-38.1351, -69.8585) -> (-37.8902, -68.4523)
  line L26 (-37.9483, -62.8561) -> (-36.102, -62.8561)
  constraint horizontal L3
  constraint collinear L5 L6
  constraint collinear L13 L14
  constraint parallel L17 L21
  constraint parallel L21 L22
  constraint coincident L3 L24.start
  constraint parallel L3 L24
  constraint horizontal L26
extrude "Extrude36" cut sketch "Sketch65" along normal blind 0.8 bodies 3
move_body "Move8" bodies 3 to x (-1, 0, 0) y (0, 1, 0) z (0, 0, -1) at (0.1352, 55, 17)
move_body "Move9" bodies 3 to x (1, 0, 0) y (0, 1, 0) z (0, 0, 1) at (-1.1352, 1, -3.5)
sketch "Sketch66" plane through (0, 0, 13.5) normal (0, 0, 1) x (-1, 0, 0)
  line L0 (43.1, 21.3) -> (-42.1, 21.3)
  line L1 (-43.1, 20.3) -> (-43.1, -20.3)
  line L2 (-42.1, -21.3) -> (43.1, -21.3)
  line L3 (44.1, -20.3) -> (44.1, 20.3)
  line L4 (-0.9865, 8.952) -> (-0.8228, 18.3259)
  line L5 (-1.216, 18.3813) -> (-3.937, 8.2519)
  line L6 (-5.4673, 8.1893) -> (-2.8485, 19.7453)
  line L7 (-4.7939, 20.0201) -> (-5.2938, 20.0289)
  line L8 (-5.3297, 19.8702) -> (-7.9485, 8.3142)
  line L9 (-10.0025, 8.1092) -> (-12.0022, 8.1441)
  line L10 (-7.7934, 20.0725) -> (-8.2933, 20.0812)
  line L11 (-7.2935, 20.0638) -> (-6.7936, 20.055)
  line L12 (-6.8479, 19.8152) -> (-9.4667, 8.2591)
  line L13 (-11.0024, 8.1267) -> (-11.5023, 8.1354)
  line L14 (-11.2523, 8.131) -> (-11.5023, 8.1354)
  line L15 (-9.5026, 8.1005) -> (-11.7563, 8.1398)
  line L16 (-9.5026, 8.1005) -> (-12.0022, 8.1441)
  line L17 (-9.3291, 19.9401) -> (-11.9479, 8.384)
  line L18 (-13.0731, 10.0629) -> (-10.8473, 19.885)
  line L19 (-13.31, 19.1686) -> (-13.4681, 10.1106)
  line L20 (-3.7473, 8) -> (-2.0038, 7.9696)
  line L21 (-7.7569, 8.07) -> (-5.6658, 8.0335)
  line L22 (-3.0401, 19.9895) -> (-5.1312, 20.026)
  line L23 (-7.0395, 20.0593) -> (-9.1306, 20.0958)
  line L24 (-11.0389, 20.1291) -> (-12.2927, 20.151)
  line L25 (-12.0022, 8.1441) -> (-9.6652, 8.1033)
  arc A0 (-2.0038, 7.9696) -> (-0.9865, 8.952) centre (-1.9863, 8.9694) ccw
  arc A1 (-12.2927, 20.151) -> (-13.31, 19.1686) centre (-12.3102, 19.1512) ccw
  arc A2 (-3.937, 8.2519) -> (-3.7473, 8) centre (-3.7438, 8.2) ccw
  arc A3 (-0.8228, 18.3259) -> (-1.216, 18.3813) centre (-1.0228, 18.3294) ccw
  arc A4 (-5.6658, 8.0335) -> (-5.4673, 8.1893) centre (-5.6623, 8.2335) ccw
  arc A5 (-7.9485, 8.3142) -> (-7.7569, 8.07) centre (-7.7534, 8.27) ccw
  arc A6 (-2.8485, 19.7453) -> (-3.0401, 19.9895) centre (-3.0436, 19.7895) ccw
  arc A7 (-5.1312, 20.026) -> (-5.3297, 19.8702) centre (-5.1347, 19.826) ccw
  arc A8 (-6.8479, 19.8152) -> (-7.0395, 20.0593) centre (-7.043, 19.8594) ccw
  arc A9 (-9.1306, 20.0958) -> (-9.3291, 19.9401) centre (-9.1341, 19.8959) ccw
  arc A10 (-9.6652, 8.1033) -> (-9.4667, 8.2591) centre (-9.6617, 8.3033) ccw
  arc A11 (-11.9479, 8.384) -> (-11.7563, 8.1398) centre (-11.7528, 8.3398) ccw
  arc A12 (-10.8473, 19.885) -> (-11.0389, 20.1291) centre (-11.0424, 19.9292) ccw
  arc A13 (-13.4681, 10.1106) -> (-13.0731, 10.0629) centre (-13.2682, 10.1071) ccw
  line L26 (-38.15, 14.4) -> (-37.3598, 11.0378)
  line L27 (-37.3598, 11.0378) -> (-39.189, 11.6451)
  line L28 (-39.189, 11.6451) -> (-38.4793, 14.6952)
  line L29 (-38.4793, 14.6952) -> (-38.15, 14.4)
  line L30 (-37.4517, 10.761) -> (-37.7923, 6.8561)
  line L31 (-37.7923, 6.8561) -> (-39.35, 11.1)
  line L32 (-39.35, 11.1) -> (-39.2554, 11.3599)
  line L33 (-39.2554, 11.3599) -> (-37.4517, 10.761)
  line L34 (-41.1421, 17.5164) -> (-38.6549, 15.2689)
  line L35 (-38.6549, 15.2689) -> (-39.4312, 11.9335)
  line L36 (-39.4312, 11.9335) -> (-41.1421, 17.5164)
  line L37 (-36.8902, 12.4523) -> (-37.1351, 13.8585)
  line L38 (-37.1351, 13.8585) -> (-34.6232, 13.8585)
  line L39 (-34.6232, 13.8585) -> (-32.75, 19.5)
  line L40 (-32.75, 19.5) -> (-30.5, 19.5)
  line L41 (-30.5, 19.5) -> (-35.102, 6.8561)
  line L42 (-35.102, 6.8561) -> (-36.9483, 6.8561)
  line L43 (-36.9483, 6.8561) -> (-35.0902, 12.4523)
  line L44 (-35.0902, 12.4523) -> (-36.8902, 12.4523)
  line L45 (-38.8305, 15.8426) -> (-41.3179, 18.0901)
  line L46 (-41.3179, 18.0901) -> (-41.75, 19.5)
  line L47 (-41.75, 19.5) -> (-39.95, 19.5)
  line L48 (-39.95, 19.5) -> (-38.8305, 15.8426)
  arc A14 (-42.1, 21.3) -> (-43.1, 20.3) centre (-42.1, 20.3) ccw
  arc A15 (-43.1, -20.3) -> (-42.1, -21.3) centre (-42.1, -20.3) ccw
  arc A16 (43.1, -21.3) -> (44.1, -20.3) centre (43.1, -20.3) ccw
  arc A17 (44.1, 20.3) -> (43.1, 21.3) centre (43.1, 20.3) ccw
  dimension "d212" = 1
  dimension "d213" = 0.2
  constraint parallel L6 L8
  constraint midpoint L9 L13.start
  constraint midpoint L13 L14.start
  constraint parallel L9 L15
  constraint parallel L17 L18
  constraint collinear L23 L24
  constraint tangent L20 A0
  constraint tangent L4 A0
  constraint tangent L24 A1
  constraint tangent L19 A1
  constraint equal A0 A1
  constraint tangent L5 A2
  constraint tangent L20 A2
  constraint tangent L4 A3
  constraint tangent L5 A3
  constraint equal A2 A3
  constraint tangent L6 A4
  constraint tangent L21 A4
  constraint equal A2 A4
  constraint tangent L8 A5
  constraint tangent L21 A5
  constraint equal A2 A5
  constraint tangent L6 A6
  constraint tangent L22 A6
  constraint equal A2 A6
  constraint coincident L7.end L22
  constraint coincident L7.end L8
  constraint tangent L22 A7
  constraint tangent L8 A7
  constraint equal A2 A7
  constraint coincident L11.end L12
  constraint coincident L11.end L23
  constraint tangent L12 A8
  constraint tangent L23 A8
  constraint equal A2 A8
  constraint tangent L17 A9
  constraint tangent L23 A9
  constraint equal A2 A9
  constraint coincident L15.start L12
  constraint coincident L15.start L25
  constraint tangent L12 A10
  constraint tangent L25 A10
  constraint equal A2 A10
  constraint coincident L9.end L15
  constraint coincident L9.end L17
  constraint tangent L15 A11
  constraint tangent L17 A11
  constraint equal A2 A11
  constraint tangent L24 A12
  constraint tangent L18 A12
  constraint equal A2 A12
  constraint tangent L18 A13
  constraint tangent L19 A13
  constraint equal A2 A13
  measures "d212" radius of A0
  measures "d213" radius of A2
move_body "Move10" bodies 3 to x (1, 0, 0) y (0, -1, 0) z (0, 0, -1) at (0, -60.6, 13.5)
move_body "Move11" bodies 3 to x (1, 0, 0) y (0, 1, 0) z (0, 0, 1) at (0, 5, 0)
move_face "OffsetFaces1" offset -1 1 faces at (-43.5, -7, 3.3333) on bodies 1
sketch "Sketch71" plane through (-44.5, 0, 0) normal (1, 0, 0) x (0, 1, 0)
  line L0 (20.3, 11) -> (-20.3, 11)
  line L1 (-20.3, 4) -> (-21, 4)
  line L2 (-21, 4) -> (-21, 2)
  line L3 (-21, 2) -> (21, 2)
  line L4 (21, 2) -> (21, 4)
  line L5 (-20.3, 11) -> (-10, 11)
  line L6 (-10, 11) -> (-10, 10)
  line L7 (-10, 10) -> (-20.3, 10)
  line L8 (-20.3, 10) -> (-20.3, 11)
  line L9 (20.3, 11) -> (10, 11)
  line L10 (10, 11) -> (10, 10)
  line L11 (10, 10) -> (20.3, 10)
  line L12 (20.3, 10) -> (20.3, 11)
  line L13 (-10, 10) -> (11, 10)
  line L14 (11, 10) -> (11, 8)
  line L15 (11, 8) -> (-10, 8)
  line L16 (-10, 8) -> (-10, 10)
  line L17 (-20.3, 11) -> (-20.3, 4)
  line L18 (21, 4) -> (20.3, 4)
  line L19 (20.3, 4) -> (20.3, 11)
  dimension "d248" = 10.3
  dimension "d249" = 1
  dimension "d250" = 10.3
  dimension "d251" = 1
  dimension "d252" = 2
  constraint horizontal L5
  constraint vertical L6
  constraint horizontal L7
  constraint vertical L8
  constraint coincident L0.end L5.start
  constraint horizontal L9
  constraint vertical L10
  constraint horizontal L11
  constraint vertical L12
  constraint coincident L0.start L9.start
  constraint horizontal L13
  constraint vertical L14
  constraint horizontal L15
  constraint vertical L16
  measures "d248" distance of L0.end L5.end
  measures "d249" distance of L0.end L7.end
  measures "d250" distance of L0.start L9.end
  measures "d251" distance of L0.start L11.end
  measures "d252" distance of L6.end L15.end
extrude "Extrude41" cut sketch "Sketch71" against normal blind 1 draft -45 contours L11 L13 L14 L15 L16 bodies 1
sketch "Sketch72" plane through (-44.5, 0, 0) normal (1, 0, 0) x (0, 1, 0)
  line L0 (11, 10) -> (11, 8)
  line L1 (11, 8) -> (-10, 8)
  line L2 (-10, 8) -> (-10, 10)
  line L3 (-10, 10) -> (11, 10)
  line L4 (20.3, 11) -> (-20.3, 11)
  line L5 (-20.3, 4) -> (-21, 4)
  line L6 (-21, 4) -> (-21, 2)
  line L7 (-21, 2) -> (21, 2)
  line L8 (21, 2) -> (21, 4)
  line L9 (-21, 4) -> (21, 4)
  line L10 (21, 4) -> (21, 2)
  line L11 (21, 2) -> (-21, 2)
  line L12 (-21, 2) -> (-21, 4)
  line L13 (-20.3, 11) -> (-20.3, 4)
  line L14 (21, 4) -> (20.3, 4)
  line L15 (20.3, 4) -> (20.3, 11)
  constraint horizontal L9
  constraint vertical L10
  constraint horizontal L11
  constraint vertical L12
  constraint coincident L7.end L8.start
  constraint coincident L5.end L6.start
extrude "Extrude42" add sketch "Sketch72" along normal blind 0.7 contours L5 L6 L7 L8 L9 L10 L11 L12 L14 bodies 1
move_face "OffsetFaces2" offset 1 1 faces at (38.5972, 13.7, 3) on bodies 1
move_face "OffsetFaces3" offset 1 1 faces at (36.6706, 15.5, 3) on bodies 1
move_face "OffsetFaces4" offset 0.2 1 faces at (4.1333, 8, 3.3333) on bodies 1
move_face "OffsetFaces5" offset 0.2 1 faces at (33.7765, 22.2333, 9.65) on bodies 1